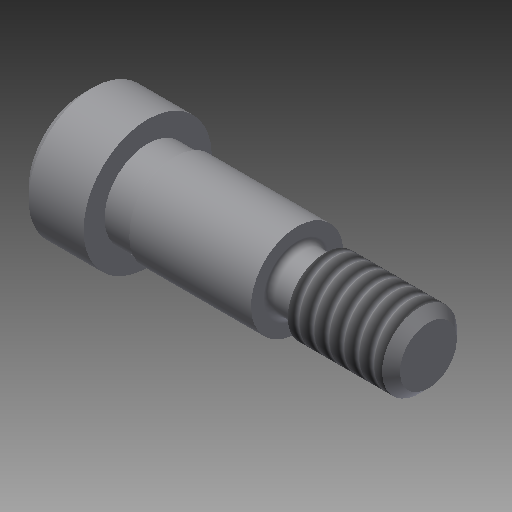
# Autodesk Inventor part: 2281_b
Saved by Autodesk Inventor 2019 (Build 230136000, 136)
## iProperties
Category: PARTsolutions
Company: 8020
Created: 2019-11-08
Part Number: 2281_b
Material: Generic
Catalog Web Link: www.cadenas.de
Description: 2281, 2282, 2280, 2290_b-Roller Wheels
Vendor: 8020
Document SubType Name: Modeling
Designer: psadmin
Manufacturer: 8020
Mass: 1.41262 g
Surface Area: 8.99428 cm^2
Volume: 1.41262 cm^3
Density: 1 g/cm^3
Appearance: PSOLRGB-192-192-192
PSOL_IDENT_0: {$CADENAS_DATA\23d-libs\8020\inch\linear_motion\2281_bolt.prj},175 {VTYP=3D},{NB=2281_b},{LINA=2281_
PSOL_IDENT_1: b},{NN=2281, 2282, 2280, 2290_b},{DATE=01.10.2019 06:04:24},{GEOMDATE=01.03.2012 00:00:00},{VERSION=
PSOL_IDENT_2: },{LINEID=10},{WBVAR=BT,RI},{WBNUMERIC=}  {NB=2281_b},{LINA=2281_b},{KT=DUMMY},{PN=2281},{NO=1},{MAT=
PSOL_IDENT_3: Self-lubricating, fiberglass-reinforced black nylon.},{BT=2},{BT1= '2','Permanent Lubricated Bronze
PSOL_IDENT_4: Bushing' },{MT=10 Series},{RI=10},{RI1= '10','10 Series','15','15 Series' },{A=1.500},{B=1.125},{C=0
PSOL_IDENT_5: .240},{D=0.480},{E=0.563},{F=0.188},{G=0.314},{H=0.214},{J=0.118},{K=0.622},{L=0.429},{M=0.320},{N=1
PSOL_IDENT_6: /4-20},{N1=0.2500},{P=0.060},{Q=0.378},{W=.070},{G1=0.375},{K1=0.000},{NTP=3382},{FT=0.087}
NN: 2281, 2282, 2280, 2290_b
NT: Roller Wheels
NB: 2281_b
NBSYN: $PN._b
LINA: 2281_b
PN: 2281
MAT: Self-lubricating, fiberglass-reinforced black nylon.
BT: Permanent Lubricated Bronze Bushing
MT: 10 Series
RI: 10 Series
A: 1.5
B: 1.125
C: 0.24
D: 0.48
E: 0.563
F: 0.188
G: 0.314
H: 0.214
J: 0.118
K: 0.622
L: 0.429
M: 0.32
N: 1/4-20
P: 0.06
Q: 0.378
W: .070
NTP: 3382
FT: 0.087
SUPPLIER: 8020
ARTICLENO: 2281_b
BOMINFO: 2281_b
CREATOR: CADENAS GmbH
Title: 2281_b
Author: Cadenas PARTsolutions
Comments: Roller Wheels
Autodesk Inventor part; units mm, degrees
sketch "Sketch_1" plane through (0, 0, 0) normal (0, 0, 1) x (1, 0, 0)
  line L0 (23.8252, 0) -> (-5.4356, 0)
  line L1 (-5.4356, 0) -> (-5.4356, 4.6863)
  line L2 (-5.4356, 4.6863) -> (-4.6736, 5.4483)
  line L3 (-4.6736, 5.4483) -> (0, 5.4483)
  line L4 (0, 5.4483) -> (0, 3.6703)
  line L5 (0, 3.6703) -> (2.1082, 3.6703)
  arc A0 (2.1082, 3.6703) -> (2.3622, 3.9243) centre (2.1082, 3.9243) ccw
  line L6 (2.3622, 3.9243) -> (12.7, 3.9243)
  line L7 (12.7, 3.9243) -> (12.7, 2.8702)
  arc A1 (12.7, 2.8702) -> (13.208, 2.3622) centre (13.208, 2.8702) ccw
  line L8 (13.208, 2.3622) -> (14.8082, 2.3622)
  arc A2 (14.8082, 2.3622) -> (15.0622, 2.6162) centre (14.8082, 2.6162) ccw
  line L9 (15.0622, 2.6162) -> (15.0622, 3.175)
  line L10 (15.0622, 3.175) -> (23.0695, 3.175)
  line L11 (23.0695, 3.175) -> (23.8252, 2.4194)
  line L12 (23.8252, 2.4194) -> (23.8252, 0)
  line L13 (23.8252, 0) -> (-5.4356, 0)
  constraints: 28 end point, 6 point on circle, 3 centre point
revolve "Revolution1" add sketch "Sketch_1" angle 360 about axis through (23.8252, 0, 0) along (1, 0, 0)
thread "Thread1" size "1/4-20 UNC" class "2A" standard "ANSI Unified Screw Threads" full length
ref_plane "bolt_XY" through (0, 0, 0) normal (1, 0, 0) x (0, 0, -1)
ref_plane "bolt_YZ" through (0, 0, 0) normal (0, 0, -1) x (0, 1, 0)
ref_plane "bolt_ZX" through (0, 0, 0) normal (0, 1, 0) x (1, 0, 0)
ref_plane "bolt1_XY" through (15.6972, 0, 0) normal (1, 0, 0) x (0, 0, -1)
ref_plane "bolt1_YZ" through (15.6972, 0, 0) normal (0, 0, -1) x (0, 1, 0)
ref_plane "bolt1_ZX" through (15.6972, 0, 0) normal (0, 1, 0) x (1, 0, 0)
body "Solid1"
